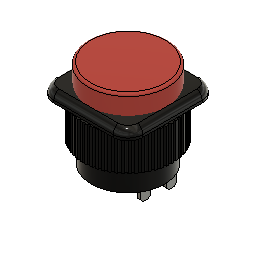
Momentary Push Button - Red v2 (Autodesk Fusion 360 design; units mm, degrees)
Autodesk Fusion 360 part; units mm, degrees
note: some values were not read from the file. Set by a fixed rule: which sketch regions a step uses.
sketch "Sketch1" plane through (0, 0, 0) normal (0, 1, 0) x (1, 0, 0)
  line L0 (6, -9) -> (-6, -9)
  line L1 (-9, -6) -> (-9, 6)
  line L2 (-6, 9) -> (6, 9)
  line L3 (9, 6) -> (9, -6)
  arc A0 (9, 6) -> (6, 9) centre (6, 6) ccw
  line L4 (0, 9) -> (0, -9) construction
  arc A1 (-6, 9) -> (-9, 6) centre (-6, 6) ccw
  arc A2 (6, -9) -> (9, -6) centre (6, -6) ccw
  arc A3 (-9, -6) -> (-6, -9) centre (-6, -6) ccw
  circle A4 centre (0, 0) radius 8
  line L5 (-9, 0) -> (9, 0) construction
  circle A5 centre (0, 0) radius 8.5
  dimension "d3" = 3
  dimension "d4" = 16
  dimension "d14" = 18
  dimension "d15" = 18
  dimension "d16" = 3
  dimension "d17" = 3
  dimension "d25" = 17
  constraint perpendicular L0 L1
  constraint parallel L0 L2
  constraint parallel L1 L3
  constraint horizontal L0
  constraint coincident A4.centre A5.centre
  constraint tangent L3 A0
  constraint symmetric L2.end L4 L2.start
  constraint symmetric A0 L4 A1
  constraint coincident L2 L4.start
  constraint tangent L2 A1
  constraint tangent L1 A3
  constraint tangent L3 A2
  constraint coincident A3 L0.end
  constraint coincident L0 L4.end
  constraint coincident A2 L3.end
  constraint tangent L0 A2
  constraint tangent L0 A3
  constraint coincident L0.start A2.start
  constraint coincident L0.end A3.end
  constraint coincident L1.start A3.start
  constraint tangent L1 A1
  constraint midpoint L1 L5.start
  constraint midpoint L3 L5.end
  constraint midpoint L4 A4.centre
  constraint concentric A4 A5
  measures "d3" radius of A0
  measures "d4" diameter of A4
  measures "d14" distance of L1 L3
  measures "d15" distance of L0 L2
  measures "d16" radius of A2
  measures "d17" radius of A3
  measures "d25" diameter of A5
sketch "Sketch2" plane through (0, 0, 0) normal (1, 0, 0) x (0, 0, -1)
  line L0 (0, 0) -> (0, 2)
  line L1 (0, 2) -> (-8, 2)
  line L2 (6, 0) -> (-6, 0) construction
  line L3 (-8, 2) -> (-8, 0) construction
  line L4 (-8, 2) -> (-8, 0.6646) construction
  line L5 (0, 0.5) -> (-9, 0.5) construction
  line L6 (-6, 0) -> (0, 0)
  line L7 (0, 0) -> (-9, 0)
  line L8 (-9, 0) -> (-9, 0.5)
  arc A0 (-8, 2) -> (-9, 0.5) centre (-7.375, 0.5) ccw
  dimension "d10" = 2
  dimension "d11" = 8
  dimension "d12" = 0.5
  dimension "d18" = 9
  constraint coincident L0.start L6.end
  constraint coincident L0 L1.start
  constraint perpendicular L0 L1
  constraint horizontal L1
  constraint coincident L2 L3.end
  constraint perpendicular L2 L3
  constraint coincident L1 L3.start
  constraint perpendicular L1 L4
  constraint coincident L3 L4.end
  constraint coincident L0 L5.start
  constraint perpendicular L3 L5
  constraint perpendicular L0 L7
  constraint tangent L8 A0
  measures "d10" distance of L1 L2
  measures "d11" distance of L0 L3
  measures "d12" distance of L2 L5
  measures "d18" distance of L0.start L7.end
sweep "Sweep1" add profiles "Sketch2" path "Sketch1" along L0 A3 L1 A1 L2 A0 L3 A2 section 1 makes body 1
extrude "Extrude1" add sketch "Sketch1" along normal blind 6.3 separate body contours A4 makes body 2 in component "Button"
fillet "Fillet1" radius 0.5 1 edges at (-7.4586, 6.3, 2.8929) on bodies 2 in component "Button"
extrude "Extrude1'" add sketch "Sketch1" against normal blind 0.5 separate body contours A5 makes body 3 in component "Shaft Spacer"
sketch "Sketch1 (2)" plane through (0, -0.5, 0) normal (0, -1, 0) x (1, 0, 0) in component "Shaft"
  circle A0 centre (0, 0) radius 9
  circle A1 centre (0, 0) radius 7.4
  dimension "d29" = 18
  dimension "d32" = 14.8
  constraint concentric A0 A1
  measures "d29" diameter of A0
  measures "d32" diameter of A1
extrude "Extrude1''" add sketch "Sketch1 (2)" along normal blind 11.5 separate body contours A1 makes body 4 in component "Shaft"
extrude "Extrude1'''" add sketch "Sketch1 (2)" along normal blind 7 separate body makes body 5 in component "Retaining Ring"
sketch "Sketch1 (3)" plane through (0, -7.5, 0) normal (0, -1, 0) x (1, 0, 0) in component "Retaining Ring"
  circle A0 centre (0, 0) radius 7.4
  circle A1 centre (0, 0) radius 9
  circle A2 centre (0, 9) radius 0.25
  line L0 (0, 0) -> (0, 12) construction
  dimension "d44" = 0.5
  constraint coincident A1 A2.centre
  constraint coincident A0.centre A1.centre
  constraint vertical L0
  constraint coincident A2.centre L0
  measures "d44" diameter of A2
extrude "Extrude2" cut sketch "Sketch1 (3)" against normal blind 7 contours A1 A2 picked at (-0.0062, 8.9166) bodies 5 in component "Retaining Ring"
pattern_circular "C-Pattern1" count 58 over 360 about axis through (0, 1.75, 0) along (0, 1, 0) of "Extrude2" in component "Retaining Ring"
sketch "Sketch1 (4)" plane through (0, -12, 0) normal (0, -1, 0) x (1, 0, 0) in component "Connections"
  circle A0 centre (0, 0) radius 7.4
  line L0 (0, 0) -> (0, 9) construction
  line L1 (0, 9) -> (0, 0) construction
  line L2 (0, 0) -> (0, -9) construction
  line L3 (0, 0) -> (9, 0) construction
  line L4 (0, 0) -> (-9, 0) construction
  line L5 (-2.8, 0.2001) -> (-2.2, 0.2001)
  line L6 (-2.2, 0.2001) -> (-2.2, -1.7999)
  line L7 (-2.2, -1.7999) -> (-2.8, -1.7999)
  line L8 (-2.8, -1.7999) -> (-2.8, 0.2001)
  line L9 (2.2, 0.2001) -> (2.2, -1.7999)
  line L10 (2.8, 0.2001) -> (2.2, 0.2001)
  line L11 (2.8, -1.7999) -> (2.8, 0.2001)
  line L12 (2.2, -1.7999) -> (2.8, -1.7999)
  line L13 (-2.5, 0.2001) -> (-2.5, -1.7999) construction
  line L14 (-3.3, -4.5041) -> (-2.7, -4.5041)
  line L15 (-2.7, -4.5041) -> (-2.7, -6.5041)
  line L16 (-2.7, -6.5041) -> (-3.3, -6.5041)
  line L17 (-3.3, -6.5041) -> (-3.3, -4.5041)
  line L18 (3.3, -6.5041) -> (3.3, -4.5041)
  line L19 (2.7, -4.5041) -> (2.7, -6.5041)
  line L20 (2.7, -6.5041) -> (3.3, -6.5041)
  line L21 (3.3, -4.5041) -> (2.7, -4.5041)
  line L22 (-3, -4.5041) -> (-3, -6.5041) construction
  dimension "d35" = 2
  dimension "d36" = 0.6
  dimension "d37" = 2.5
  dimension "d38" = 0.6
  dimension "d39" = 2
  dimension "d40" = 3
  constraint coincident A0.centre L0.start
  constraint vertical L0
  constraint parallel L0 L2
  constraint perpendicular L0 L3
  constraint perpendicular L1 L4
  constraint horizontal L5
  constraint vertical L6
  constraint horizontal L7
  constraint vertical L8
  constraint symmetric L1 L5.start L10.start
  constraint symmetric L1 L5.end L9.start
  constraint symmetric L1 L6.end L9.end
  constraint symmetric L1 L7.end L11.start
  constraint midpoint L5 L13.start
  constraint midpoint L7 L13.end
  constraint horizontal L14
  constraint vertical L15
  constraint horizontal L16
  constraint vertical L17
  constraint symmetric L2 L14.start L18.end
  constraint symmetric L2 L14.end L19.start
  constraint symmetric L2 L15.end L19.end
  constraint symmetric L2 L16.end L18.start
  constraint midpoint L14 L22.start
  constraint midpoint L16 L22.end
  measures "d35" distance of L5.start L7.end
  measures "d36" distance of L5.start L5.end
  measures "d37" distance of L2 L13
  measures "d38" distance of L14.start L14.end
  measures "d39" distance of L14.start L16.end
  measures "d40" distance of L2 L22
extrude "Extrude1''''" add sketch "Sketch1 (4)" along normal blind 5.5 separate body contours L5 L6 L7 L8 | L9 L10 L11 L12 | L14 L15 L16 L17 | L18 L19 L20 L21 makes body 6 at (2.8, -13.8333, -1.1332) makes body 7 at (2.7, -13.8333, -5.1707) makes body 8 at (-2.2, -13.8333, -0.4666) makes body 9 at (-2.7, -13.8333, -5.1707) in component "Connections"
chamfer "Chamfer1" distance 0.5 angle 45 8 edges at (-2.5, -17.5, 0.2001) (-2.5, -17.5, -1.7999) (3, -17.5, -4.5041) (3, -17.5, -6.5041) (2.5, -17.5, 0.2001) (2.5, -17.5, -1.7999) (-3, -17.5, -4.5041) (-3, -17.5, -6.5041) on bodies 6 7 8 9 in component "Connections"
copy_body "Body->Comp1" bodies 1 removing the originals makes body 10 in component "Top"
component "Button" placed x (1, 0, 0) y (0, 1, 0) z (0, 0, 1) at (0, -0.5, 0)
component "Shaft Spacer" placed x (1, 0, 0) y (0, 1, 0) z (0, 0, 1) at (0, 0, 0)
component "Shaft" placed x (1, 0, 0) y (0, 1, 0) z (0, 0, 1) at (0, 0, 0)
component "Connections" placed x (1, 0, 0) y (0, 1, 0) z (0, 0, 1) at (0, 0, 0)
component "Top" placed x (1, 0, 0) y (0, 1, 0) z (0, 0, 1) at (0, 0, 0)
component "Retaining Ring" placed x (1, 0, 0) y (0, 1, 0) z (0, 0, 1) at (0, 0, 0) in component "Shaft"
